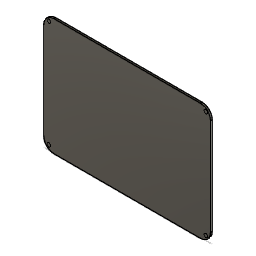
Bandeja Feldherr Tapa (Autodesk Fusion 360 design; units mm, degrees)
Autodesk Fusion 360 part; units mm, degrees
sketch "Base" plane through (0, 0, 0) normal (0, 0, 1) x (1, 0, 0)
  line L0 (0, 0) -> (245, 0)
  line L1 (245, 0) -> (245, -172)
  line L2 (245, -172) -> (0, -172)
  line L3 (0, -172) -> (0, 0)
  circle A0 centre (15, -15) radius 15
  circle A1 centre (230, -15) radius 15
  circle A2 centre (15, -157) radius 15
  circle A3 centre (230, -157) radius 15
  dimension "d4" = 172
  dimension "d5" = 245
  dimension "d6" = 30
  dimension "d7" = 30
  dimension "d8" = 30
  dimension "d9" = 30
  constraint horizontal L0
  constraint vertical L1
  constraint horizontal L2
  constraint vertical L3
  constraint coincident L0.start L3.end
  constraint tangent L0 A0
  constraint tangent L3 A0
  constraint tangent L0 A1
  constraint tangent L1 A1
  constraint tangent L1 A3
  constraint tangent L2 A3
  constraint tangent L2 A2
  constraint tangent L3 A2
  measures "d4" distance of L0.start L2.end
  measures "d5" distance of L0.start L0.end
  measures "d6" diameter of A0
  measures "d7" diameter of A1
  measures "d8" diameter of A2
  measures "d9" diameter of A3
extrude "Extrude1" add sketch "Base" along normal blind 2.5 contours L0 L1 L2 L3 A0 A1 A2 A3 | A0 | A1 | A2 | A3
sketch "Pared" plane through (0, 0, 2.5) normal (0, 0, 1) x (1, 0, 0)
  arc A0 (15, 0) -> (0, -15) centre (15, -15) ccw
  line L0 (0, -15) -> (0, -157)
  arc A1 (0, -157) -> (15, -172) centre (15, -157) ccw
  line L1 (15, -172) -> (230, -172)
  arc A2 (230, -172) -> (245, -157) centre (230, -157) ccw
  line L2 (245, -157) -> (245, -15)
  arc A3 (245, -15) -> (230, 0) centre (230, -15) ccw
  line L3 (230, 0) -> (15, 0)
  line L4 (2, -2) -> (243, -2)
  line L5 (243, -2) -> (243, -170)
  line L6 (243, -170) -> (2, -170)
  line L7 (2, -170) -> (2, -2)
  circle A4 centre (15, -157) radius 13
  circle A5 centre (15, -15) radius 13
  circle A6 centre (230, -15) radius 13
  circle A7 centre (230, -157) radius 13
  line L8 (0, 0) -> (15, -15) construction
  line L9 (4.3934, -4.3934) -> (5.8076, -5.8076) construction
  line L10 (243, -2) -> (230, -15) construction
  line L11 (243, -2) -> (258.3137, -2) construction
  line L12 (240.6066, -4.3934) -> (239.1924, -5.8076) construction
  line L13 (243, -170) -> (230, -157) construction
  line L14 (243, -170) -> (258.3137, -170) construction
  line L15 (240.6066, -167.6066) -> (239.1924, -166.1924) construction
  line L16 (2, -170) -> (15, -157) construction
  line L17 (2, -170) -> (14.3137, -170) construction
  line L18 (4.3934, -167.6066) -> (5.8076, -166.1924) construction
  dimension "d12" = 2
  dimension "d13" = 2
  dimension "d14" = 2
  dimension "d15" = 2
  dimension "d53" = 2
  dimension "d55" = 135
  dimension "d56" = 2
  dimension "d57" = 135
  dimension "d58" = 2
  dimension "d59" = 45
  dimension "d60" = 2
  constraint horizontal L4
  constraint vertical L5
  constraint horizontal L6
  constraint vertical L7
  constraint tangent L7 A4
  constraint tangent L4 A5
  constraint tangent L4 A6
  constraint tangent L5 A7
  constraint tangent L7 A5
  constraint tangent L5 A6
  constraint tangent L6 A7
  constraint tangent L6 A4
  constraint coincident L8.start origin
  constraint coincident A0.centre A5.centre
  constraint coincident A0 L9.start
  constraint coincident A5 L9.end
  constraint collinear L8 L9
  constraint horizontal L11
  constraint coincident A3.centre A6.centre
  constraint coincident A3 L12.start
  constraint coincident A6 L12.end
  constraint collinear L10 L12
  constraint horizontal L14
  constraint coincident A2.centre A7.centre
  constraint coincident A2 L15.start
  constraint coincident A7 L15.end
  constraint collinear L13 L15
  constraint horizontal L17
  constraint coincident A1.centre A4.centre
  constraint coincident A1 L18.start
  constraint coincident A4 L18.end
  constraint collinear L16 L18
  measures "d12" distance of L3 L4
  measures "d13" distance of L0 L7
  measures "d14" distance of L1 L6
  measures "d15" distance of L2 L5
  measures "d53" distance of L9.start L9.end
  measures "d55" angle of L10 L11
  measures "d56" distance of L12.start L12.end
  measures "d57" angle of L13 L14
  measures "d58" distance of L15.start L15.end
  measures "d59" angle of L16 L17
  measures "d60" distance of L18.start L18.end
sketch "Imanes" plane through (0, 0, 0) normal (0, 0, -1) x (-1, 0, 0)
  circle A0 centre (-7.2218, -7.2218) radius 4
  circle A1 centre (-15, -15) radius 15 construction
  line L0 (0, 0) -> (-15, -15) construction
  circle A2 centre (-7.2218, -7.2218) radius 2.6
  circle A3 centre (-7.2218, -164.7782) radius 4
  circle A4 centre (-237.7782, -164.7782) radius 4
  circle A5 centre (-237.7782, -7.2218) radius 4
  circle A6 centre (-230, -15) radius 15 construction
  circle A7 centre (-230, -157) radius 15 construction
  circle A8 centre (-15, -157) radius 15 construction
  line L1 (0, -172) -> (-15, -157) construction
  line L2 (-245, -172) -> (-230, -157) construction
  line L3 (-245, 0) -> (-230, -15) construction
  circle A9 centre (-237.7782, -7.2218) radius 2.6
  circle A10 centre (-237.7782, -164.7782) radius 2.6
  circle A11 centre (-7.2218, -164.7782) radius 2.6
  point P0 (0, -172)
  point P1 (-245, -172)
  point P2 (-245, 0)
  dimension "d32" = 8
  dimension "d33" = 5.2
  dimension "d43" = 8
  dimension "d44" = 8
  dimension "d45" = 8
  dimension "d46" = 5.2
  dimension "d47" = 5.2
  dimension "d48" = 5.2
  constraint tangent A0 A1
  constraint coincident L0.start origin
  constraint coincident A1.centre L0.end
  constraint concentric A0 A2
  constraint tangent A5 A6
  constraint tangent A3 A8
  constraint coincident P0 L1.start
  constraint coincident A8.centre L1.end
  constraint coincident P1 L2.start
  constraint coincident A7.centre L2.end
  constraint coincident P2 L3.start
  constraint coincident A6.centre L3.end
  constraint coincident A5.centre L3
  constraint concentric A5 A9
  constraint coincident A4.centre L2
  constraint concentric A4 A10
  constraint coincident A0.centre L0
  constraint concentric A3 A11
  constraint coincident L1 A3.centre
  constraint tangent A4 A7
  measures "d32" diameter of A0
  measures "d33" diameter of A2
  measures "d43" diameter of A3
  measures "d44" diameter of A4
  measures "d45" diameter of A5
  measures "d46" diameter of A9
  measures "d47" diameter of A10
  measures "d48" diameter of A11
extrude "Extrude6" cut sketch "Imanes" against normal blind 2 contours A2 | A9 | A10 | A11
equation "d4 = bandeja_y"
equation "d5 = bandeja_x"
equation "d6 = bandeja_filet"
equation "d7 = bandeja_filet"
equation "d8 = bandeja_filet"
equation "d9 = bandeja_filet"
equation "d10 = extrusion_bandeja_piso"
equation "d12 = bandeja_pared"
equation "d13 = bandeja_pared"
equation "d14 = bandeja_pared"
equation "d15 = bandeja_pared"
equation "d32 = iman_pared"
equation "d33 = iman_diametro"
equation "d37 = -extrusion_iman_inferior"
equation "d43 = iman_pared"
equation "d44 = iman_pared"
equation "d45 = iman_pared"
equation "d46 = iman_diametro"
equation "d47 = iman_diametro"
equation "d48 = iman_diametro"
equation "d53 = bandeja_pared"
equation "d56 = bandeja_pared"
equation "d58 = bandeja_pared"
equation "d60 = bandeja_pared"
equation "bandeja_x = 245 mm"
equation "bandeja_y = 172 mm"
equation "bandeja_filet = 30 mm"
equation "bandeja_pared = 2 mm"
equation "iman_diametro = 5.2 mm"
equation "iman_pared = iman_diametro + 2.8 mm"
equation "extrusion_bandeja_piso = 2.5 mm"
equation "extrusion_iman_inferior = 2 mm"
named bodies: "Bandeja Feldherr Tapa"
